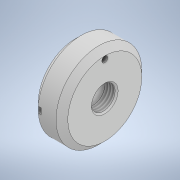
# Autodesk Inventor part: 711137
Saved by Autodesk Inventor 2022 (Build 260153000, 153)
## iProperties
Created: 2021-10-22
Part Number: 711137
Material: Типовые
Document SubType Name: Modeling
Designer: RaNSiD
Density: 1 g/cm^3
Appearance: По умолчанию
Author: RaNSiD
Autodesk Inventor part; units mm, degrees
ref_plane "YZ Plane" through (0, 0, 0) normal (1, 0, 0) x (0, 1, 0)
ref_plane "XZ Plane" through (0, 0, 0) normal (0, 1, 0) x (-1, 0, 0)
ref_plane "XY Plane" through (0, 0, 0) normal (0, 0, 1) x (1, 0, 0)
sketch "Эскиз5" plane through (0, 0, 0) normal (0, 0, 1) x (1, 0, 0)
  line L0 (0, 0) -> (-20, 0)
  line L1 (-20, 0) -> (-20, 25)
  line L2 (-16, 29) -> (-4, 29)
  line L3 (0, 25) -> (0, 0)
  line L4 (-4, 29) -> (0, 25)
  line L5 (-16, 29) -> (-20, 25)
  point P0 (-20, 29)
  point P1 (0, 29)
  dimension "d35" = 20
  dimension "d36" = 29
  dimension "d37" = 4
  dimension "d38" = 4
  dimension "d39" = 4
  dimension "d40" = 4
  constraints: 12 end point, 4 point on line, 2 parallel, 1 horizontal, 1 perpendicular
  measures "d35" distance of point (-20, 29) point (0, 29)
  measures "d36" distance of L0.end point (-20, 29)
  measures "d37" distance of L2.end point (0, 29)
  measures "d38" distance of L3.start point (0, 29)
  measures "d39" distance of L2.start point (-20, 29)
  measures "d40" distance of L1.end point (-20, 29)
revolve "Вращение3" add sketch "Эскиз5" angle 360 about axis through (0, 0, 0) along (-1, 0, 0)
sketch "Эскиз6" plane through (0, 0, 0) normal (1, 0, 0) x (0, 0, -1)
  line L0 (0, 0) -> (0, 23) construction
  dimension "d42" = 23
  constraints: 2 end point, 1 coincident, 1 vertical
  measures "d42" distance of L0.start L0.end
hole "Отверстие2" at (0, 23, 0) direction (-1, 0, 0) diameter 4 depth 4
sketch "Эскиз7" plane through (0, 0, 0) normal (1, 0, 0) x (0, 0, -1)
  point P0 (0, 0)
  point P1 (0, 0)
  constraints: 1 coincident
hole "Отверстие3" at (0, 0, 0) direction (-1, 0, 0) diameter 16 depth 8 tip angle 140 countersink diameter 18 countersink angle 90
sketch "Эскиз8" plane through (0, 0, 0) normal (0, 0, 1) x (1, 0, 0)
  line L0 (-20, -25) -> (-20, 25) construction
  line L1 (-20, 2) -> (-14, 2)
  line L2 (-14, 2) -> (-14, -2)
  line L3 (-14, -2) -> (-20, -2)
  line L4 (-20, -2) -> (-20, 2)
  point P0 (0, 0)
  point P1 (-20, 0)
  point P2 (-20, 0)
  dimension "d57" = 6
  dimension "d58" = 4
  constraints: 8 end point, 2 midpoint, 2 parallel, 1 coincident, 1 horizontal, 1 perpendicular, 1 point on line
  measures "d57" distance of L2.end L3.end
  measures "d58" distance of L1.end L2.end
extrude "Выдавливание2" cut sketch "Эскиз8" along normal through all both and the other way through all
thread "Резьба3" size "M16x2" class "6H" standard "ANSI Metric M Profile" full length
equation "\"d38\" = d37"
equation "\"d39\" = d37"
equation "\"d40\" = d39"
